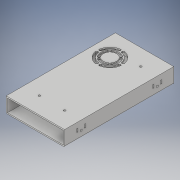
# Autodesk Inventor part: LRS-350
Saved by Autodesk Inventor 2019 (Build 230136000, 136)
## iProperties
Created: 2020-11-04
Part Number: LRS-350
Material: Generic
Document SubType Name: Modeling
Designer: Brendan
Density: 1 g/cm^3
Appearance: Default
Author: Brendan
Autodesk Inventor part; units mm, degrees
ref_plane "YZ Plane" through (0, 0, 0) normal (1, 0, 0) x (0, 1, 0)
ref_plane "XZ Plane" through (0, 0, 0) normal (0, 1, 0) x (-1, 0, 0)
ref_plane "XY Plane" through (0, 0, 0) normal (0, 0, 1) x (1, 0, 0)
sketch "Sketch1" plane through (0, 0, 0) normal (0, 0, 1) x (1, 0, 0)
  line L0 (0, 0) -> (115, 0)
  line L1 (115, 0) -> (115, 30)
  line L2 (115, 30) -> (0, 30)
  line L3 (0, 30) -> (0, 0)
  dimension "d0" = 115
  dimension "d1" = 30
  constraints: 8 end point, 2 parallel, 1 horizontal, 1 perpendicular
  measures "d0" distance of L2.end L1.end
  measures "d1" distance of L1.end L0.end
extrude "Extrusion1" add sketch "Sketch1" along normal blind 215
sketch "Sketch2" plane through (115, 0, 0) normal (1, 0, 0) x (0, 0, -1)
  line L0 (-215, 0) -> (-215, 30) projected
  circle A0 centre (-182.5, 12.5) radius 2
  point P0 (0, 0)
  dimension "d6" = 4
  constraints: 1 centre point
  measures "d6" diameter of A0
extrude "Extrusion2" cut sketch "Sketch2" against normal blind 215
sketch "Sketch3" plane through (115, 0, 0) normal (1, 0, 0) x (0, 0, -1)
  line L0 (0, 30) -> (0, 0) projected
  circle A0 centre (-32.5, 12.5) radius 2
  dimension "d11" = 4
  constraints: 1 centre point
  measures "d11" diameter of A0
extrude "Extrusion3" cut sketch "Sketch3" against normal blind 215
sketch "Sketch4" plane through (0, 30, 0) normal (0, 1, 0) x (1, 0, 0)
  line L0 (115, 0) -> (115, -215) projected
  circle A0 centre (32.5, -182.0659) radius 2
  circle A1 centre (82.5, -182.5) radius 2
  point P0 (0, 0)
  dimension "d18" = 4
  dimension "d19" = 4
  constraints: 2 centre point
  measures "d18" diameter of A0
  measures "d19" diameter of A1
extrude "Extrusion4" cut sketch "Sketch4" against normal blind 215
sketch "Sketch5" plane through (0, 30, 0) normal (0, 1, 0) x (1, 0, 0)
  circle A0 centre (32.5, -32.5) radius 2
  circle A1 centre (82.5, -32.5) radius 2
  point P0 (115, 0)
  dimension "d26" = 4
  constraints: 2 centre point
  measures "d26" diameter of A0
extrude "Extrusion5" cut sketch "Sketch5" against normal blind 215
sketch "Sketch6" plane through (115, 0, 0) normal (1, 0, 0) x (0, 0, -1)
  line L0 (0, 0) -> (-215, 0) projected
  line L1 (-176, 12.8) -> (-174, 12.8)
  line L2 (-174, 12.8) -> (-174, 19.7)
  line L3 (-174, 19.7) -> (-176, 19.7)
  line L4 (-176, 19.7) -> (-176, 12.8)
  line L5 (-189, 19.7) -> (-189, 12.8)
  line L6 (-176, 12.8) -> (-176, 19.7)
  line L7 (-189, 12.8) -> (-191, 12.8)
  line L8 (-191, 12.8) -> (-191, 19.7)
  line L9 (-191, 19.7) -> (-189, 19.7)
  line L10 (-189, 19.7) -> (-189, 12.8)
  dimension "d34" = 2
  dimension "d35" = 6.9
  dimension "d36" = 13
  dimension "d38" = 2
  constraints: 20 end point, 5 parallel, 2 horizontal, 2 perpendicular
  measures "d34" distance of L3.end L2.end
  measures "d35" distance of L2.end L1.end
  measures "d36" distance of L6.start L5.end
  measures "d38" distance of L8.end L9.end
extrude "Extrusion6" cut sketch "Sketch6" against normal blind 215
sketch "Sketch7" plane through (115, 0, 0) normal (1, 0, 0) x (0, 0, -1)
  line L0 (-39, 12.5) -> (-39, 12.8)
  line L1 (-39, 12.8) -> (-41, 12.8)
  line L2 (-41, 12.8) -> (-41, 19.7)
  line L3 (-41, 19.7) -> (-39, 19.7)
  line L4 (-39, 19.7) -> (-39, 12.8)
  line L5 (-26, 19.7) -> (-26, 12.8)
  line L6 (-39, 12.8) -> (-39, 19.7)
  line L7 (-26, 12.8) -> (-24, 12.8)
  line L8 (-24, 12.8) -> (-24, 19.7)
  line L9 (-24, 19.7) -> (-26, 19.7)
  line L10 (-26, 19.7) -> (-26, 12.8)
  point P0 (0, 0)
  point P1 (-32.5, 12.5)
  dimension "d51" = 2
  dimension "d55" = 2
  constraints: 22 end point, 5 parallel, 2 horizontal, 2 perpendicular
  measures "d51" distance of L2.end L3.end
  measures "d55" distance of L9.end L8.end
extrude "Extrusion7" cut sketch "Sketch7" against normal blind 215
sketch "Sketch8" plane through (0, 30, 0) normal (0, 1, 0) x (1, 0, 0)
  line L0 (0, 0) -> (115, 0) projected
  line L1 (0, 0) -> (36.7, 0)
  line L2 (0, -47.45) -> (0, 0)
  line L3 (36.7, -47.45) -> (35.2, -47.45)
  line L4 (38.2, -47.45) -> (35.2, -47.45)
  line L5 (38.2, -24.7179) -> (38.2, -25.7302)
  line L6 (35.2, -25.7302) -> (35.2, -24.7179)
  line L7 (14.9802, -45.95) -> (13.9679, -45.95)
  line L8 (14.9802, -48.95) -> (13.9679, -48.95)
  line L9 (35.2, -69.1698) -> (35.2, -70.1821)
  line L10 (38.2, -69.1698) -> (38.2, -70.1821)
  line L11 (59.4321, -45.95) -> (58.4198, -45.95)
  line L12 (59.4321, -48.95) -> (58.4198, -48.95)
  arc A0 (32.8957, -22.7412) -> (11.9912, -43.6457) centre (36.7, -47.45) ccw
  arc A1 (33.5182, -27.7047) -> (16.9547, -44.2682) centre (36.7, -47.45) ccw
  arc A2 (16.9547, -50.6318) -> (33.5182, -67.1953) centre (36.7, -47.45) ccw
  arc A3 (11.9912, -51.2543) -> (32.8957, -72.1588) centre (36.7, -47.45) ccw
  arc A4 (40.5043, -72.1588) -> (61.4088, -51.2543) centre (36.7, -47.45) ccw
  arc A5 (61.4088, -43.6457) -> (40.5043, -22.7412) centre (36.7, -47.45) ccw
  arc A6 (39.8818, -67.1953) -> (56.4453, -50.6318) centre (36.7, -47.45) ccw
  arc A7 (56.4453, -44.2682) -> (39.8818, -27.7047) centre (36.7, -47.45) ccw
  arc A8 (56.4453, -44.2682) -> (58.4198, -45.95) centre (58.4198, -43.95) ccw
  arc A9 (59.4321, -45.95) -> (61.4088, -43.6457) centre (59.4321, -43.95) ccw
  arc A10 (58.4198, -48.95) -> (56.4453, -50.6318) centre (58.4198, -50.95) ccw
  arc A11 (61.4088, -51.2543) -> (59.4321, -48.95) centre (59.4321, -50.95) ccw
  arc A12 (35.2, -69.1698) -> (33.5182, -67.1953) centre (33.2, -69.1698) ccw
  arc A13 (32.8957, -72.1588) -> (35.2, -70.1821) centre (33.2, -70.1821) ccw
  arc A14 (38.2, -70.1821) -> (40.5043, -72.1588) centre (40.2, -70.1821) ccw
  arc A15 (39.8818, -67.1953) -> (38.2, -69.1698) centre (40.2, -69.1698) ccw
  arc A16 (13.9679, -48.95) -> (11.9912, -51.2543) centre (13.9679, -50.95) ccw
  arc A17 (16.9547, -50.6318) -> (14.9802, -48.95) centre (14.9802, -50.95) ccw
  arc A18 (11.9912, -43.6457) -> (13.9679, -45.95) centre (13.9679, -43.95) ccw
  arc A19 (14.9802, -45.95) -> (16.9547, -44.2682) centre (14.9802, -43.95) ccw
  arc A20 (35.2, -24.7179) -> (32.8957, -22.7412) centre (33.2, -24.7179) ccw
  arc A21 (33.5182, -27.7047) -> (35.2, -25.7302) centre (33.2, -25.7302) ccw
  arc A22 (38.2, -25.7302) -> (39.8818, -27.7047) centre (40.2, -25.7302) ccw
  arc A23 (40.5043, -22.7412) -> (38.2, -24.7179) centre (40.2, -24.7179) ccw
  line L13 (36.7, -47.45) -> (55.0141, -47.45) construction
  line L14 (36.7, -47.45) -> (54.7, -47.45) construction
  line L15 (36.7, -47.45) -> (54.7, -47.45) construction
  line L16 (36.7, -47.45) -> (54.7, -47.45) construction
  line L17 (36.7, -47.45) -> (54.7, -47.45) construction
  line L18 (25.1699, -58.3154) -> (25.8945, -57.6107)
  line L19 (27.2078, -56.3334) -> (27.2201, -56.3456)
  line L20 (26.6533, -58.3173) -> (25.9412, -59.0381)
  line L21 (23.6943, -35.0158) -> (23.2849, -35.4486)
  line L22 (26.5971, -36.5903) -> (25.8963, -35.862)
  line L23 (46.8054, -58.1779) -> (47.5501, -58.8729)
  line L24 (47.5118, -57.5547) -> (48.2283, -58.2712)
  line L25 (45.8924, -38.2576) -> (46.3924, -38.2576) construction
  line L26 (46.8047, -36.6382) -> (47.5212, -35.9217)
  line L27 (45.8924, -38.2576) -> (46.3924, -38.2576) construction
  line L28 (47.5118, -37.3453) -> (48.2283, -36.6288)
  line L29 (25.2306, -36.6124) -> (25.9352, -37.3446)
  arc A24 (22.1757, -36.8178) -> (22.1599, -58.0607) centre (36.7, -47.45) ccw
  arc A25 (23.6896, -35.011) -> (23.2849, -35.4486) centre (36.7, -47.45) ccw
  arc A26 (26.1215, -39.8939) -> (26.1267, -55.0134) centre (36.7, -47.45) ccw
  arc A27 (47.2829, -32.8897) -> (26.1672, -32.8534) centre (36.7, -47.45) ccw
  arc A28 (44.2318, -36.8541) -> (29.1932, -36.8364) centre (36.7, -47.45) ccw
  arc A29 (29.2259, -58.0866) -> (44.2754, -58.0147) centre (36.7, -47.45) ccw
  arc A30 (47.2959, -54.9818) -> (47.2959, -39.9182) centre (36.7, -47.45) ccw
  arc A31 (26.1969, -62.068) -> (47.3712, -61.9457) centre (36.7, -47.45) ccw
  arc A32 (51.2603, -58.0329) -> (51.2603, -36.8671) centre (36.7, -47.45) ccw
  arc A33 (47.5118, -37.3453) -> (47.2959, -39.9182) centre (48.926, -38.7595) ccw
  arc A34 (51.2603, -36.8671) -> (48.2283, -36.6288) centre (49.6425, -38.043) ccw
  arc A35 (44.2318, -36.8541) -> (46.8047, -36.6382) centre (45.3905, -35.224) ccw
  arc A36 (47.5212, -35.9217) -> (47.2829, -32.8897) centre (46.107, -34.5075) ccw
  arc A37 (26.1672, -32.8534) -> (25.8963, -35.862) centre (27.3375, -34.4753) ccw
  arc A38 (26.5971, -36.5903) -> (29.1932, -36.8364) centre (28.0383, -35.2036) ccw
  arc A39 (26.1215, -39.8939) -> (25.9352, -37.3446) centre (24.494, -38.7314) ccw
  arc A40 (25.2306, -36.6124) -> (22.1757, -36.8178) centre (23.7895, -37.9992) ccw
  arc A41 (22.1599, -58.0607) -> (25.1699, -58.3154) centre (23.7755, -56.8817) ccw
  arc A42 (25.8945, -57.6107) -> (26.1267, -55.0134) centre (24.5, -56.177) ccw
  arc A43 (25.9412, -59.0381) -> (26.1969, -62.068) centre (27.3639, -60.4438) ccw
  arc A44 (29.2259, -58.0866) -> (26.6533, -58.3173) centre (28.076, -59.723) ccw
  arc A45 (47.3712, -61.9457) -> (47.5501, -58.8729) centre (46.1855, -60.3351) ccw
  arc A46 (46.8054, -58.1779) -> (44.2754, -58.0147) centre (45.4408, -59.6401) ccw
  arc A47 (47.2959, -54.9818) -> (47.5118, -57.5547) centre (48.926, -56.1405) ccw
  arc A48 (48.2283, -58.2712) -> (51.2603, -58.0329) centre (49.6425, -56.857) ccw
  point P0 (35.2, -22.495)
  point P1 (38.2, -27.5063)
  point P2 (38.2, -22.495)
  point P3 (35.2, -27.5063)
  point P4 (16.7563, -45.95)
  point P5 (16.7563, -48.95)
  point P6 (11.745, -48.95)
  point P7 (35.2, -72.405)
  point P8 (38.2, -72.405)
  point P9 (56.6437, -45.95)
  point P10 (61.655, -45.95)
  point P11 (61.655, -48.95)
  point P12 (11.745, -45.95)
  point P13 (56.6437, -48.95)
  point P14 (35.2, -67.3937)
  point P15 (38.2, -67.3937)
  point P16 (23.6235, -59.8195)
  point P17 (27.9191, -57.0362)
  point P18 (24.4031, -60.5948)
  point P19 (49.1943, -60.4074)
  point P20 (24.4005, -34.3076)
  point P21 (45.532, -37.9109)
  point P22 (27.1607, -38.6182)
  point P23 (49.7766, -35.0805)
  point P24 (49.0695, -34.3734)
  point P25 (46.2391, -38.618)
  point P26 (46.2391, -56.282)
  point P27 (45.5318, -56.9894)
  point P28 (49.7766, -59.8195)
  point P29 (27.8679, -37.9109)
  constraints: 130 point on circle, 64 tangent, 58 end point, 49 centre point, 34 point on line, 29 equal radius, 8 horizontal, 3 coincident, 1 parallel, 1 perpendicular
sketch "Sketch9" plane through (0, 0, 215) normal (0, 0, 1) x (1, 0, 0)
  line L0 (0, 30) -> (0, 0) projected
  line L1 (115, 0) -> (115, 30) projected
  line L2 (2.5, 27.5) -> (112.5, 27.5)
  line L3 (112.5, 27.5) -> (112.5, 2.5)
  line L4 (112.5, 2.5) -> (2.5, 2.5)
  line L5 (2.5, 2.5) -> (2.5, 27.5)
  constraints: 8 end point, 2 parallel, 1 horizontal, 1 perpendicular
extrude "Extrusion8" cut sketch "Sketch9" against normal blind 212.5
extrude "Extrusion9" cut sketch "Sketch8" against normal blind 5
fillet "Fillet1" radius 2 1 edges at (115, 0, 107.5)
fillet "Fillet2" radius 2 1 edges at (0, 0, 107.5)
body "Solid1"
